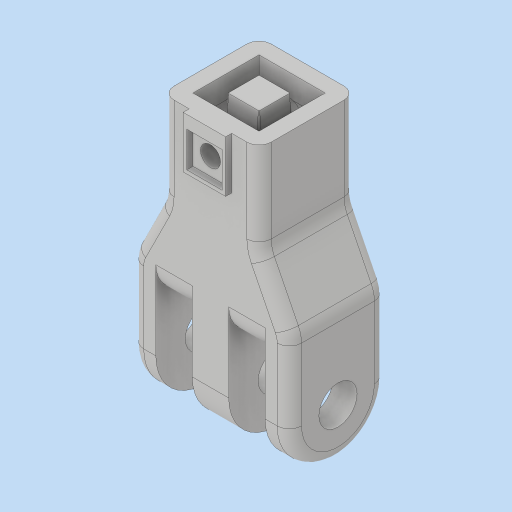
# Autodesk Inventor part: aret-rodtop-fork
Saved by Autodesk Inventor 2024 (Build 280153000, 153)
## iProperties
Created: 2022-10-05
Part Number: aret-rodtop-fork
Material: Generic
Document SubType Name: Modeling
Designer: Karbosch
Mass: 9.9452 g
Surface Area: 60.7469 cm^2
Volume: 9.9452 cm^3
Density: 1 g/cm^3
Appearance: Default
Author: Karbosch
Autodesk Inventor part; units mm, degrees
ref_plane "YZ Plane" through (0, 0, 0) normal (1, 0, 0) x (0, 1, 0)
ref_plane "XZ Plane" through (0, 0, 0) normal (0, 1, 0) x (-1, 0, 0)
ref_plane "XY Plane" through (0, 0, 0) normal (0, 0, 1) x (1, 0, 0)
sketch "Sketch115" plane through (0, 0, 0) normal (0, 1, 0) x (-1, 0, 0)
  line L0 (-4.9167, 4.9167) -> (4.9167, -4.9167) construction
  line L1 (4.9167, 4.9167) -> (-4.9167, -4.9167) construction
  line L2 (-2.85, 2.85) -> (2.85, 2.85)
  line L3 (2.85, 2.85) -> (2.85, -2.85)
  line L4 (2.85, -2.85) -> (-2.85, -2.85)
  line L5 (-2.85, -2.85) -> (-2.85, 2.85)
  line L6 (-3.925, 3.925) -> (3.925, -3.925) construction
  line L7 (3.925, 3.925) -> (-3.2901, -3.2901) construction
  line L8 (5.15, 5.15) -> (-5.15, 5.15)
  line L9 (-5.15, 5.15) -> (-5.15, -5.15)
  line L10 (-5.15, -5.15) -> (5.15, -5.15)
  line L11 (5.15, -5.15) -> (5.15, 5.15)
  line L12 (8, 8) -> (-8, 8)
  line L13 (-8, 8) -> (-8, -8)
  line L14 (-8, -8) -> (8, -8)
  line L15 (8, -8) -> (8, 8)
  line L16 (0, 0) -> (-2, 0)
  line L17 (-2, 0) -> (-1, 1.7321)
  line L18 (-1, 1.7321) -> (1, 1.7321)
  line L19 (1, 1.7321) -> (2, 0)
  line L20 (2, 0) -> (1, -1.7321)
  line L21 (1, -1.7321) -> (-1, -1.7321)
  line L22 (-1, -1.7321) -> (-2, 0)
  dimension "d539" = 5.7
  dimension "d540" = 10.3
  dimension "d541" = 16
  dimension "d667" = 2
  constraints: 46 end point, 6 parallel, 4 horizontal, 3 perpendicular, 2 midpoint, 1 coincident, 13 other
  measures "d539" distance of L3.end L4.end
  measures "d540" distance of L10.end L9.end
  measures "d541" distance of L14.end L13.end
  measures "d667" distance of L16.start L16.end
extrude "Extrusion85" add sketch "Sketch115" along normal blind 25
sketch "Sketch135" plane through (0, 0, 0) normal (0, -1, 0) x (1, 0, 0)
  line L0 (-8, -8) -> (-8, 8) projected
  line L1 (-8, 8) -> (6, 8)
  line L2 (6, 8) -> (6, -6)
  line L3 (6, -6) -> (-8, -6)
  line L4 (-8, -6) -> (-8, 8)
  point P0 (0, 0)
  constraints: 8 end point, 2 parallel, 1 horizontal, 1 perpendicular
extrude "Extrusion100" add sketch "Sketch135" against normal blind 5
ref_plane "Work Plane56" through (0, 0, -8) normal (0, 0, 1) x (1, 0, 0)
ref_plane "Work Plane58" through (16.9697, -2.8756, 0) normal (0, 1, 0) x (-1, 0, 0)
ref_plane "Work Plane59" through (-8, 25, 0) normal (1, 0, 0) x (0, 1, 0)
sketch "Sketch140" plane through (-8, 25, 0) normal (1, 0, 0) x (0, 1, 0)
  line L0 (-20, -2.85) -> (-20, 2.85) projected
  line L1 (-20, 2.85) -> (-20, -2.85) projected
  line L2 (-20, 5.15) -> (-20, -5.15) projected
  line L3 (-20, -5.15) -> (-20, 5.15) projected
  line L4 (-20, -5.15) -> (-20, 5.15) projected
  circle A0 centre (-5, 0) radius 1.6
  point P0 (-25, 0)
  dimension "d658" = 3.2
  constraints: 1 centre point
  measures "d658" diameter of A0
sketch "Sketch141" plane through (-8, 25, 0) normal (1, 0, 0) x (0, 1, 0)
  line L0 (-2.1, 2.9) -> (-7.9, 2.9)
  line L1 (-7.9, 2.9) -> (-7.9, -2.9)
  line L2 (-7.9, -2.9) -> (-2.1, -2.9)
  line L3 (-2.1, -2.9) -> (-2.1, 2.9)
  line L4 (-2.1, 2.9) -> (-7.9, -2.9) construction
  line L5 (-7.9, 2.9) -> (-2.1, -2.9) construction
  line L6 (-1.5, 3.5) -> (-8.5, 3.5)
  line L7 (-8.5, 3.5) -> (-8.5, -3.5)
  line L8 (-8.5, -3.5) -> (-1.5, -3.5)
  line L9 (-1.5, 3.5) -> (-8.5, -3.5) construction
  line L10 (-8.5, 3.5) -> (-1.5, -3.5) construction
  line L11 (-1.5, 3.5) -> (0, 3.5)
  line L12 (0, 3.5) -> (0, -3.5)
  line L13 (0, -3.5) -> (-1.5, -3.5)
  point P0 (-25, 0)
  point P1 (-5, 0)
  dimension "d668" = 5.8
  dimension "d669" = 5.8
  dimension "d670" = 7
  dimension "d671" = 7
  constraints: 28 end point, 4 midpoint, 4 perpendicular, 3 horizontal, 3 parallel
  measures "d668" distance of L2.end L1.end
  measures "d669" distance of L1.end L0.end
  measures "d670" distance of L8.end L7.end
  measures "d671" distance of L7.end L6.end
sketch "Sketch142" plane through (0, 5, 0) normal (0, 1, 0) x (1, 0, 0)
  line L0 (1, -1.7321) -> (-1, -1.7321) projected
  line L1 (2, 0) -> (1, -1.7321) projected
  line L2 (1, 1.7321) -> (2, 0) projected
  line L3 (-1, 1.7321) -> (1, 1.7321) projected
  line L4 (-2, 0) -> (-1, 1.7321) projected
  line L5 (-1, -1.7321) -> (-2, 0) projected
  point P0 (0, 0)
extrude "Extrusion107" add sketch "Sketch142" along normal blind 5
sketch "Sketch144" plane through (0, 25, 0) normal (0, 1, 0) x (1, 0, 0)
  line L0 (1, -1.7321) -> (-1, -1.7321) projected
  line L1 (2, 0) -> (1, -1.7321) projected
  line L2 (1, 1.7321) -> (2, 0) projected
  line L3 (-1, 1.7321) -> (1, 1.7321) projected
  line L4 (-2, 0) -> (-1, 1.7321) projected
  line L5 (-1, -1.7321) -> (-2, 0) projected
  point P0 (0, 0)
extrude "Extrusion108" add sketch "Sketch144" against normal blind 2
chamfer "Chamfer19" distance 1.15 angle 70 8 edges at (0, 5, 5.15) (-5.15, 5, 0) (0, 5, -5.15) (5.15, 5, 0) (0, 5, -2.85) (2.85, 5, 0) (0, 5, 2.85) (-2.85, 5, 0) measured on face at (4.65, 5, 0) measured on face at (0, 5, -4.65) measured on face at (-3.35, 5, 0) measured on face at (0, 5, -3.35) measured on face at (-4.65, 5, 0) measured on face at (0, 5, 3.35) measured on face at (3.35, 5, 0) measured on face at (0, 5, 4.65)
ref_plane "Work Plane60" through (0, 0, 0) normal (0, 0, 1) x (1, 0, 0)
sketch "Sketch145" plane through (0, 0, 0) normal (0, 0, 1) x (1, 0, 0)
  line L0 (-8, 0) -> (-8, 25) projected
  line L1 (-8, 10) -> (-13, 0)
  line L2 (-13, 0) -> (-13, -21)
  line L3 (-13, -21) -> (-9, -21)
  line L4 (-9, -21) -> (-9, -5)
  line L5 (-9, -5) -> (-3, -5)
  line L6 (-3, -5) -> (-3, -21)
  line L7 (-3, -21) -> (0, -21)
  line L8 (0, -21) -> (0, 10)
  line L9 (-1, 10) -> (1, 10) projected
  line L10 (-8, 10) -> (0, 10)
  line L11 (8, 10) -> (13, 0)
  line L12 (13, 0) -> (13, -21)
  line L13 (13, -21) -> (9, -21)
  line L14 (9, -21) -> (9, -5)
  line L15 (9, -5) -> (3, -5)
  line L16 (3, -5) -> (3, -21)
  line L17 (3, -21) -> (0, -21)
  line L18 (1, 10) -> (-1, 10)
  line L19 (8, 10) -> (0, 10)
  line L20 (8, 0) -> (-8, 0) projected
  line L21 (3, -5) -> (8, 0)
  line L22 (8, 0) -> (-8, 0)
  line L23 (-8, 0) -> (-3, -5)
  point P0 (0, 0)
  dimension "d686" = 4
  dimension "d688" = 6
  constraints: 42 end point, 10 symmetric about line, 4 perpendicular, 2 horizontal, 1 collinear, 1 midpoint, 1 point on line, 1 vertical
  measures "d686" distance of L2.end L3.end
  measures "d688" distance of L4.end L5.end
extrude "Extrusion109" add sketch "Sketch145" along normal mid plane 16
fillet "Fillet6" radius 8 6 edges at (0, -21, -8) (0, -21, 8) (11, -21, 8) (11, -21, -8) (-11, -21, 8) (-11, -21, -8)
fillet "Fillet8" radius 0.4 4 edges at (2.85, 17.5, -2.85) (-2.85, 17.5, -2.85) (-2.85, 17.5, 2.85) (2.85, 17.5, 2.85)
move faces "Move6" translate (0, -8, 0) faces at (4.3833, 10, 0.8167)
chamfer "Chamfer24" distance 1.15 angle 70 12 edges at (-2.85, 2, 0) (-2.7328, 2, 2.7328) (0, 2, 2.85) (2.7328, 2, 2.7328) (2.85, 2, 0) (2.7328, 2, -2.7328) (0, 2, -2.85) (-2.7328, 2, -2.7328) (0, 2, 5.15) (-5.15, 2, 0) (0, 2, -5.15) (5.15, 2, 0) measured on face at (-4.65, 2, 0) measured on face at (-3.35, 2, 0) measured on face at (4.65, 2, 0) measured on face at (3.35, 2, 0) measured on face at (0, 2, -4.65) measured on face at (3.0864, 2, 3.0864) measured on face at (3.0864, 2, -3.0864) measured on face at (-3.0864, 2, -3.0864) measured on face at (0, 2, -3.35) measured on face at (0, 2, 3.35) measured on face at (0, 2, 4.65) measured on face at (-3.0864, 2, 3.0864)
sketch "Sketch147" plane through (-3, -13, 0) normal (-1, 0, 0) x (0, 0, 1)
  arc A0 (-8, 0) -> (8, 0) centre (0, 0) ccw projected
  circle A1 centre (0, 0) radius 3.15
  point P0 (0, 13)
  dimension "d720" = 6.3
  constraints: 1 centre point, 1 coincident
  measures "d720" diameter of A1
extrude "Extrusion111" cut sketch "Sketch147" along normal through all both and the other way through all
fillet "Fillet9" radius 5 8 edges at (6, -5, 8) (-6, -5, 8) (6, -5, -8) (-6, -5, -8) (-8, 10, 0) (-13, 0, 0) (8, 10, 0) (13, 0, 0)
chamfer "Chamfer27" distance 0.3 angle 85 4 edges at (0, 25, -5.15) (5.15, 25, 0) (0, 25, 5.15) (-5.15, 25, 0) measured on face at (0, 25, 5.65) measured on face at (0, 25, -5.65) measured on face at (5.65, 25, 0) measured on face at (-5.65, 25, 0)
ref_plane "Work Plane61" through (0, 25, 8) normal (0, 0, -1) x (-1, 0, 0)
sketch "Sketch149" plane through (0, 25, 8) normal (0, 0, -1) x (-1, 0, 0)
  line L0 (-2.9, -2.1) -> (-2.9, -7.9)
  line L1 (-2.9, -7.9) -> (2.9, -7.9)
  line L2 (2.9, -7.9) -> (2.9, -2.1)
  line L3 (2.9, -2.1) -> (-2.9, -2.1)
  line L4 (-2.9, -2.1) -> (2.9, -7.9) construction
  line L5 (-2.9, -7.9) -> (2.9, -2.1) construction
  line L6 (-3.5, -1.5) -> (-3.5, -8.5)
  line L7 (-3.5, -8.5) -> (3.5, -8.5)
  line L8 (3.5, -8.5) -> (3.5, -1.5)
  line L9 (-3.5, -1.5) -> (3.5, -8.5) construction
  line L10 (-3.5, -8.5) -> (3.5, -1.5) construction
  line L11 (-3.5, -1.5) -> (-3.5, 0)
  line L12 (-3.5, 0) -> (3.5, 0)
  line L13 (3.5, 0) -> (3.5, -1.5)
  circle A0 centre (0, -5) radius 1.65
  point P0 (-25, 0)
  dimension "d729" = 5.8
  dimension "d730" = 5.8
  dimension "d731" = 7
  dimension "d732" = 7
  dimension "d733" = 3.3
  constraints: 28 end point, 4 midpoint, 4 perpendicular, 3 parallel, 1 centre point, 1 coincident
  measures "d729" distance of L2.end L1.end
  measures "d730" distance of L1.end L0.end
  measures "d731" distance of L8.end L7.end
  measures "d732" distance of L7.end L6.end
  measures "d733" diameter of A0
sketch "Sketch150" plane through (0, 25, 8) normal (0, 0, -1) x (-1, 0, 0)
  circle A0 centre (0, -5) radius 1.65 projected
  point P0 (0, -25)
extrude "Extrusion112" cut sketch "Sketch150" along normal through all both and the other way through all
sketch "Sketch151" plane through (0, 25, 8) normal (0, 0, -1) x (-1, 0, 0)
  line L0 (2.9, -2.1) -> (-2.9, -2.1) projected
  line L1 (2.9, -7.9) -> (2.9, -2.1) projected
  line L2 (-2.9, -7.9) -> (2.9, -7.9) projected
  line L3 (-2.9, -2.1) -> (-2.9, -7.9) projected
  line L4 (-3.5, -1.5) -> (-3.5, -8.5) projected
  line L5 (-3.5, -8.5) -> (3.5, -8.5) projected
  line L6 (3.5, 0) -> (3.5, -1.5) projected
  line L7 (3.5, -8.5) -> (3.5, -1.5) projected
  line L8 (-3.5, -1.5) -> (-3.5, 0) projected
  line L9 (8, 0) -> (-8, 0) projected
  point P0 (0, -25)
extrude "Extrusion113" add sketch "Sketch151" against normal blind 1
chamfer "Chamfer28" distance 0.3 angle 85 8 edges at (-2.85, 25, 0) (-2.7328, 25, 2.7328) (0, 25, 2.85) (2.7328, 25, 2.7328) (2.85, 25, 0) (2.7328, 25, -2.7328) (0, 25, -2.85) (-2.7328, 25, -2.7328) measured on face at (-2.3793, 25, -2.3793) measured on face at (2.35, 25, 0) measured on face at (0, 25, 2.35) measured on face at (-2.3793, 25, 2.3793) measured on face at (2.3793, 25, -2.3793) measured on face at (-2.35, 25, 0) measured on face at (0, 25, -2.35) measured on face at (2.3793, 25, 2.3793)
fillet "Fillet10" radius 2 26 edges at (-8.1338, 10.0316, 8) (-10.5, 5, 8) (-12.8662, -0.0316, 8) (-13, -7.0902, 8) (-13, -18.6569, 5.6569) (-13, -21, 0) (-13, -18.6569, -5.6569) (-13, -7.0902, -8) (-12.8662, -0.0316, -8) (-10.5, 5, -8) (-8.1338, 10.0316, -8) (-8, 18.0902, -8) (-8, 18.0902, 8) (8.1338, 10.0316, 8) (10.5, 5, 8) (12.8662, -0.0316, 8) (13, -7.0902, 8) (13, -18.6569, 5.6569) (13, -21, 0) (13, -18.6569, -5.6569) (13, -7.0902, -8) (12.8662, -0.0316, -8) (10.5, 5, -8) (8.1338, 10.0316, -8) (8, 18.0902, -8) (8, 18.0902, 8)
body "Solid7"
